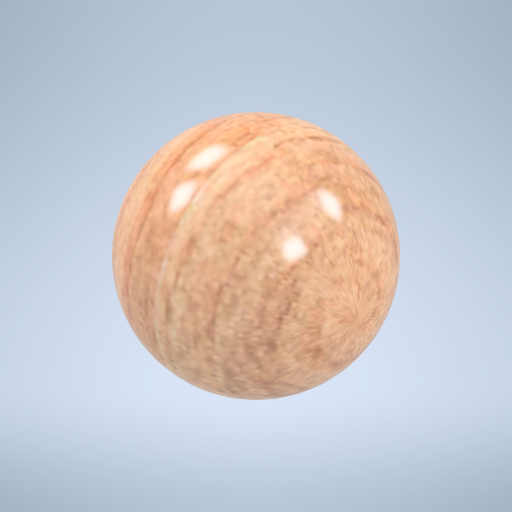
# Autodesk Inventor part: Ball
Saved by Autodesk Inventor 2023.2 (Build 272271030, 271C)
## iProperties
Created: 2022-11-29
Part Number: Ball
Material: Wood (Birch)
Document SubType Name: Modeling
Designer: kakik
Density: 0.55 g/cm^3
Appearance: Birch - Natural Polished
Author: kakik
Autodesk Inventor part; units mm, degrees
ref_plane "YZ Plane" through (0, 0, 0) normal (1, 0, 0) x (0, 1, 0)
ref_plane "XZ Plane" through (0, 0, 0) normal (0, 1, 0) x (-1, 0, 0)
ref_plane "XY Plane" through (0, 0, 0) normal (0, 0, 1) x (1, 0, 0)
sketch "Sketch1" plane through (0, 0, 0) normal (0, 1, 0) x (-1, 0, 0)
  arc A0 (-30, 0) -> (30, 0) centre (0, 0) ccw
  line L0 (30, 0) -> (-30, 0)
  dimension "d0" = 60
  constraints: 2 end point, 2 point on circle, 1 centre point, 1 coincident, 1 horizontal
  measures "d0" diameter of A0
revolve "Revolution1" add sketch "Sketch1" angle 360 about axis through (-30, 0, 0) along (1, 0, 0)
body "Solid1"
